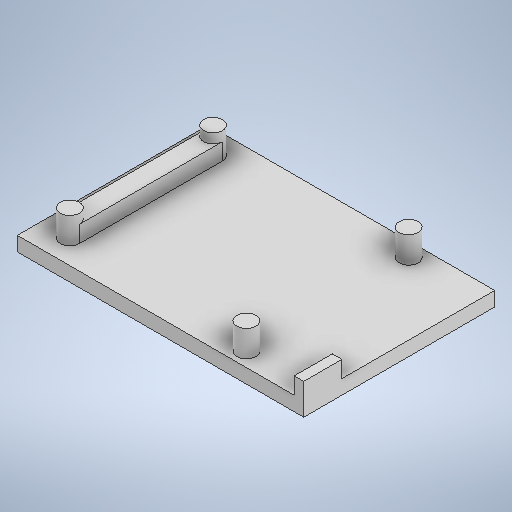
# Autodesk Inventor part: RFID Reader Frontboard
Saved by Autodesk Inventor 2025.2 (Build 292293000, 293)
## iProperties
Created: 2024-12-17
Part Number: RFID Reader Frontboard
Material: Generic
Document SubType Name: Modeling
Designer: justw
Density: 1 g/cm^3
Appearance: Default
Author: justw
Autodesk Inventor part; units mm, degrees
ref_plane "YZ Plane" through (0, 0, 0) normal (1, 0, 0) x (0, 1, 0)
ref_plane "XZ Plane" through (0, 0, 0) normal (0, 1, 0) x (-1, 0, 0)
ref_plane "XY Plane" through (0, 0, 0) normal (0, 0, 1) x (1, 0, 0)
sketch "Sketch1" plane through (0, 0, 0) normal (0, 1, 0) x (-1, 0, 0)
  line L0 (12.4084, 21.2195) -> (-47.5916, 21.2195)
  line L1 (-47.5916, 21.2195) -> (-47.5916, -18.7805)
  line L2 (-47.5916, -18.7805) -> (12.4084, -18.7805)
  line L3 (12.4084, -18.7805) -> (12.4084, 21.2195)
  circle A0 centre (6.4084, 16.2195) radius 2
  circle A1 centre (6.4084, -13.7805) radius 2
  circle A2 centre (-32.5916, 18.2195) radius 2
  circle A3 centre (-32.5916, -15.7805) radius 2
  line L4 (-47.5916, 21.2195) -> (-47.5916, 0)
  line L5 (-47.5916, 21.2195) -> (-45.5916, 21.2195)
  line L6 (-45.5916, 21.2195) -> (-45.5916, 13.2195)
  line L7 (-45.5916, 13.2195) -> (-47.5916, 13.2195)
  line L8 (-47.5916, 13.2195) -> (-47.5916, 21.2195)
  line L9 (8.4084, -15.7805) -> (4.4084, -15.7805)
  line L10 (4.4084, -15.7805) -> (4.4084, 18.2195)
  line L11 (4.4084, 18.2195) -> (8.4084, 18.2195)
  line L12 (8.4084, 18.2195) -> (8.4084, -15.7805)
  point P0 (0, 0)
  point P1 (8.4084, -13.7805)
  point P2 (8.4084, 16.2195)
  point P3 (4.4084, 16.2195)
  point P4 (4.4084, -13.7805)
  dimension "d0" = 40
  dimension "d1" = 60
  dimension "d2" = 4
  dimension "d3" = 4
  dimension "d4" = 4
  dimension "d5" = 4
  dimension "d6" = 5
  dimension "d7" = 5
  dimension "d9" = 6
  dimension "d10" = 6
  dimension "d11" = 3
  dimension "d12" = 3
  dimension "d13" = 15
  dimension "d14" = 15
  dimension "d15" = 34
  dimension "d16" = 39
  dimension "d17" = 30
  dimension "d26" = 8
  dimension "d27" = 2
  constraints: 26 end point, 6 parallel, 4 centre point, 3 horizontal, 3 perpendicular, 1 point on line
  measures "d0" distance of L2.end L0.start
  measures "d1" distance of L1.end L2.end
  measures "d2" diameter of A0
  measures "d3" diameter of A1
  measures "d4" diameter of A2
  measures "d5" diameter of A3
  measures "d6" distance from line of L0 A0.centre
  measures "d7" distance from line of L2 A1.centre
  measures "d9" distance from line of A0.centre L3
  measures "d10" distance from line of L3 A1.centre
  measures "d11" distance from line of L0 A2.centre
  measures "d12" distance from line of A3.centre L2
  measures "d13" distance from line of L1 A2.centre
  measures "d14" distance from line of A3.centre L1
  measures "d15" distance of A3.centre A2.centre
  measures "d16" horizontal distance of A2.centre A0.centre
  measures "d17" distance of A0.centre A1.centre
  measures "d26" distance of L5.end L6.end
  measures "d27" distance of L6.end L7.end
extrude "Extrusion1" add sketch "Sketch1" against normal blind 3 contours L3 L2 L1 L7 L6 L0 | L6 L7 L1 L0 | A0 | L12 A1 L10 A0 | A0 L11 L12 | A0 L10 L11 | A1 | L12 L9 A1 | A1 L9 L10 | A2 | A3
extrude "Extrusion2" add sketch "Sketch1" along normal blind 5.5 contours A0 | A1 | A2 | A3
extrude "Extrusion3" add sketch "Sketch1" along normal blind 3.5 contours L6 L7 L1 L0 | L12 A1 L10 A0
body "Solid1"
